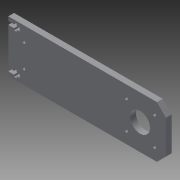
# Autodesk Inventor part: tiltColumnNonStepperSide02
Saved by Autodesk Inventor 2013 (Build 170138000, 138)
## iProperties
Created: 2014-06-14
Part Number: tiltColumnNonStepperSide02
Material: Generic
Document SubType Name: Modeling
Designer: Byron
Density: 1 g/cm^3
Author: Byron
Autodesk Inventor part; units mm, degrees
ref_plane "YZ Plane" through (0, 0, 0) normal (1, 0, 0) x (0, 1, 0)
ref_plane "XZ Plane" through (0, 0, 0) normal (0, 1, 0) x (-1, 0, 0)
ref_plane "XY Plane" through (0, 0, 0) normal (0, 0, 1) x (1, 0, 0)
sketch "Sketch1" plane through (0, 0, 0) normal (0, 0, 1) x (1, 0, 0)
  circle A0 centre (15.5, -15.5) radius 2 projected
  circle A1 centre (-15.5, -15.5) radius 2 projected
  circle A2 centre (15.5, 15.5) radius 2 projected
  circle A3 centre (-15.5, 15.5) radius 2 projected
  line L0 (-21.15, 15.4985) -> (-15.4985, 21.15) projected
  line L1 (-15.4985, 21.15) -> (15.4985, 21.15) projected
  line L2 (15.4985, 21.15) -> (21.15, 15.4985) projected
  line L3 (21.15, 15.4985) -> (21.15, -15.4985) projected
  line L4 (21.15, -15.4985) -> (15.4985, -21.15) projected
  line L5 (15.4985, -21.15) -> (-15.4985, -21.15) projected
  line L6 (-15.4985, -21.15) -> (-21.15, -15.4985) projected
  line L7 (-21.15, -15.4985) -> (-21.15, 15.4985) projected
  line L8 (28.575, -18.574) -> (28.575, 18.574)
  line L9 (28.575, 18.574) -> (18.574, 28.575)
  line L10 (18.574, 28.575) -> (-18.574, 28.575)
  line L11 (-18.574, 28.575) -> (-28.575, 18.574)
  line L12 (-28.575, 18.574) -> (-28.575, -18.574)
  line L13 (-28.575, -18.574) -> (-18.574, -28.575)
  line L14 (-18.574, -28.575) -> (18.574, -28.575)
  line L15 (18.574, -28.575) -> (28.575, -18.574)
  line L16 (-18.574, -28.575) -> (-145.574, -28.575)
  line L17 (-145.574, -28.575) -> (-145.574, 28.575)
  line L18 (-145.574, 28.575) -> (-18.574, 28.575)
  line L19 (-18.574, 28.575) -> (-18.574, -28.575)
  circle A4 centre (0, 0) radius 11 projected
  dimension "d0" = 127
  dimension "d1" = 57.15
  dimension "d2" = 57.15
  constraints: 24 end point, 2 parallel, 1 horizontal, 1 perpendicular, 7 other
  measures "d0" distance of L17.end L18.end
  measures "d1" distance between parallel lines of L10 L14
  measures "d2" distance of L16.end L17.end
extrude "Extrusion1" add sketch "Sketch1" along normal blind 6.35
sketch "Sketch2" plane through (0, 0, 6.35) normal (0, 0, 1) x (1, 0, 0)
  line L0 (-130.4486, -16.3493) -> (-130.4486, -9.9993) projected
  line L1 (-126.7402, -9.9993) -> (-126.7402, -16.3493) projected
  line L2 (-130.4486, 9.0507) -> (-130.4486, 15.4007) projected
  line L3 (-126.7402, 15.4007) -> (-126.7402, 9.0507) projected
  line L4 (-126.7402, 12.7) -> (-130.4486, 12.7) construction
  line L5 (-126.7402, -12.7) -> (-130.9009, -12.7) construction
  circle A0 centre (-128.5944, 12.7) radius 1.8542
  circle A1 centre (-128.5944, -12.7) radius 1.8542
  dimension "d5" = 3.7084
  dimension "d6" = 3.7084
  constraints: 4 end point, 2 centre point
  measures "d5" diameter of A0
  measures "d6" diameter of A1
extrude "Extrusion2" cut sketch "Sketch2" against normal through all
sketch "Sketch3" plane through (0, 0, 6.35) normal (0, 0, 1) x (1, 0, 0)
  line L0 (-145.574, -28.575) -> (-145.574, 28.575) projected
  line L1 (-151.924, 20.3708) -> (-151.924, 24.0792) projected
  line L2 (-151.924, -24.5535) -> (-151.924, -20.8451) projected
  line L3 (-131.1543, 22.225) -> (-145.574, 22.225) construction
  line L4 (-131.1543, -22.225) -> (-145.574, -22.225) construction
  line L5 (-145.574, -20.3708) -> (-132.874, -20.3708)
  line L6 (-132.874, -20.3708) -> (-132.874, -24.0792)
  line L7 (-132.874, -24.0792) -> (-145.574, -24.0792)
  line L8 (-145.574, -24.0792) -> (-145.574, -20.3708)
  line L9 (-145.574, 24.0792) -> (-132.874, 24.0792)
  line L10 (-132.874, 24.0792) -> (-132.874, 20.3708)
  line L11 (-132.874, 20.3708) -> (-145.574, 20.3708)
  line L12 (-145.574, 20.3708) -> (-145.574, 24.0792)
  line L13 (-136.43, 26.162) -> (-139.224, 26.162)
  line L14 (-139.224, 26.162) -> (-139.224, 18.288)
  line L15 (-139.224, 18.288) -> (-136.43, 18.288)
  line L16 (-136.43, 18.288) -> (-136.43, 26.162)
  line L17 (-136.43, -18.288) -> (-139.224, -18.288)
  line L18 (-139.224, -18.288) -> (-139.224, -26.162)
  line L19 (-139.224, -26.162) -> (-136.43, -26.162)
  line L20 (-136.43, -26.162) -> (-136.43, -18.288)
  dimension "d9" = 12.7
  dimension "d10" = 2.794
  dimension "d11" = 7.874
  dimension "d12" = 3.937
  dimension "d13" = 3.937
  dimension "d14" = 7.874
  dimension "d15" = 3.937
  dimension "d16" = 3.937
  dimension "d17" = 6.35
  dimension "d18" = 6.35
  dimension "d19" = 2.794
  constraints: 36 end point, 8 parallel, 6 horizontal, 4 perpendicular
  measures "d9" distance of L6.end L7.end
  measures "d10" distance of L15.end L14.end
  measures "d11" distance of L14.end L13.end
  measures "d12" distance between parallel lines of L15 L3
  measures "d13" distance between parallel lines of L13 L3
  measures "d14" distance of L19.end L17.start
  measures "d15" distance between parallel lines of L19 L4
  measures "d16" distance between parallel lines of L17 L4
  measures "d17" distance between parallel lines of L0 L14
  measures "d18" distance between parallel lines of L0 L18
  measures "d19" distance of L17.start L17.end
extrude "Extrusion3" cut sketch "Sketch3" against normal through all
equation "\"d2\" = d1"
equation "\"d12\" = d13"
equation "\"d15\" = d16"
body "Solid1"
